Autodesk Fusion 360 part; units mm, degrees
(part 3 of 3)
sketch "DownZoneCables" plane through (0, 0, -18) normal (0, 0, -1) x (1, 0, 0)
  circle A0 centre (-23.3525, 0) radius 1.55
  circle A1 centre (23.3525, 0) radius 1.55
  arc A2 (-84.3286, -41.8567) -> (-84.3286, -41.2595) centre (-82.8076, -41.5581) ccw
  arc A3 (-84.3286, -41.2595) -> (-84.3286, -41.8567) centre (-84.3576, -41.5581) ccw
  arc A4 (87.6714, -41.8567) -> (87.6714, -41.2595) centre (89.1924, -41.5581) ccw
  arc A5 (87.6714, -41.2595) -> (87.6714, -41.8567) centre (87.6424, -41.5581) ccw
  arc A6 (-84.3286, 52.7522) -> (-84.3286, 53.3494) centre (-82.8076, 53.0508) ccw
  arc A7 (-84.3286, 53.3494) -> (-84.3286, 52.7522) centre (-84.3576, 53.0508) ccw
  arc A8 (87.6714, 52.7522) -> (87.6714, 53.3494) centre (89.1924, 53.0508) ccw
  arc A9 (87.6714, 53.3494) -> (87.6714, 52.7522) centre (87.6424, 53.0508) ccw
  arc A10 (84.2133, 53.3494) -> (84.2133, 52.7522) centre (82.6924, 53.0508) ccw
  arc A11 (84.2133, 52.7522) -> (84.2133, 53.3494) centre (84.2424, 53.0508) ccw
  arc A12 (1.4807, 16.7953) -> (1.9547, 17.1586) centre (2.6428, 15.7697) ccw
  arc A13 (1.9547, 17.1586) -> (1.4807, 16.7953) centre (1.7, 17) ccw
  arc A14 (-87.7867, -41.2595) -> (-87.7867, -41.8567) centre (-89.3076, -41.5581) ccw
  arc A15 (-87.7867, -41.8567) -> (-87.7867, -41.2595) centre (-87.7576, -41.5581) ccw
  arc A16 (-1.9531, 17.1611) -> (-1.4827, 16.7932) centre (-2.655, 15.7792) ccw
  arc A17 (-1.4827, 16.7932) -> (-1.9531, 17.1611) centre (-1.7, 17) ccw
  arc A18 (-87.7753, 53.3502) -> (-87.798, 52.7535) centre (-89.3065, 53.1098) ccw
  arc A19 (-87.798, 52.7535) -> (-87.7753, 53.3502) centre (-87.7576, 53.0508) ccw
  arc A20 (84.2133, -41.2595) -> (84.2133, -41.8567) centre (82.6924, -41.5581) ccw
  arc A21 (84.2133, -41.8567) -> (84.2133, -41.2595) centre (84.2424, -41.5581) ccw
  circle A22 centre (-107.5383, -7.4166) radius 1.55
  circle A23 centre (13.049, 34.0489) radius 1.55
  circle A24 centre (13.049, -34.7379) radius 1.55
  circle A25 centre (107.424, -7.4117) radius 1.55
  circle A26 centre (-13.049, 34.0489) radius 1.55
  circle A27 centre (-13.1642, -34.387) radius 1.55
  circle A28 centre (0, 0) radius 1.55
  line L0 (139, -65) -> (139, 64.9863)
  arc A29 (139, 64.9863) -> (130.116, 73.9855) centre (130, 64.9863) ccw
  spline S0 degree 3 poles (74.4883, 73.7463) (76.9901, 72.5973) (79.4645, 71.676) (81.9056, 70.9678) (87.9623, 69.2105) (93.8091, 68.7788) (99.3307, 68.9719) (104.8445, 69.1648) (110.025, 69.9298) (114.8797, 70.7875) (120.3191, 71.7486) (125.372, 72.8483) (130.116, 73.9855) knots -1 -1 -1 -1 -0.885821 -0.885821 -0.885821 -0.602514 -0.602514 -0.602514 -0.319613 -0.319613 -0.319613 -0.002638 -0.002638 -0.002638 -0.002638
  line L1 (74.4883, 73.7463) -> (74.1645, 73.895)
  arc A30 (74.1645, 73.895) -> (73.7471, 73.9863) centre (73.7471, 72.9863) ccw
  line L2 (73.7471, 73.9863) -> (-73.8561, 73.9863)
  arc A31 (-73.8561, 73.9863) -> (-74.2689, 73.8971) centre (-73.8561, 72.9863) ccw
  line L3 (-74.2689, 73.8971) -> (-74.6062, 73.7442)
  spline S1 degree 3 poles (-130.1182, 73.9855) (-125.3557, 72.8228) (-120.2812, 71.71) (-114.815, 70.7515) (-109.9113, 69.8915) (-104.6739, 69.1384) (-99.0955, 68.9821) (-93.5592, 68.8269) (-87.6968, 69.3115) (-81.6191, 71.1146) (-79.3104, 71.7996) (-76.9712, 72.6723) (-74.6062, 73.7442) knots 0.00269 0.00269 0.00269 0.00269 0.321768 0.321768 0.321768 0.608009 0.608009 0.608009 0.892088 0.892088 0.892088 1 1 1 1
  arc A32 (-130.1182, 73.9855) -> (-139, 64.9863) centre (-130, 64.9863) ccw
  line L4 (-139, 64.9863) -> (-139, -65)
  arc A33 (-139, -65) -> (-130, -74) centre (-130, -65) ccw
  line L5 (-130, -74) -> (130, -74)
  arc A34 (130, -74) -> (139, -65) centre (130, -65) ccw
  line L6 (-0.0576, -64.1328) -> (-85.2001, -64.455) construction
  line L7 (-120.0387, -64.455) -> (-85.2001, -64.455) construction
  line L8 (-120.0387, 64.6535) -> (-120.0387, -64.455) construction
  line L9 (107.424, 64.6535) -> (-120.0387, 64.6535) construction
  line L10 (107.424, -7.4117) -> (107.424, 64.6535) construction
  line L11 (-107.5383, -58.2757) -> (-77.6055, -58.2757) construction
  line L12 (-107.5383, -54.8501) -> (-107.5383, -58.2757) construction
  line L13 (-107.5383, -7.4166) -> (-107.5383, -54.8501) construction
  line L14 (-0.0576, -58.2757) -> (-77.6055, -58.2757) construction
  line L15 (-70.0576, 34.0489) -> (-70.0576, -52.4185) construction
  line L16 (-33.1654, 34.0489) -> (-70.0576, 34.0489) construction
  line L17 (-13.049, 34.0489) -> (-33.1654, 34.0489) construction
  line L18 (-0.0576, -52.4185) -> (-70.0576, -52.4185) construction
  line L19 (-64.1025, 27.0489) -> (-64.1025, -46.5614) construction
  line L20 (-33.1654, 27.0489) -> (-64.1025, 27.0489) construction
  line L21 (13.049, 27.0489) -> (-33.1654, 27.0489) construction
  line L22 (13.049, 34.0489) -> (13.049, 27.0489) construction
  line L23 (-0.0576, -46.5614) -> (-64.1025, -46.5614) construction
  line L24 (-58.5721, 14.3434) -> (-58.5721, -40.7043) construction
  line L25 (-33.329, 14.3434) -> (-58.5721, 14.3434) construction
  line L26 (0, 0) -> (-33.329, 14.3434) construction
  line L27 (-0.0576, -40.7043) -> (-58.5721, -40.7043) construction
  line L28 (-89.3076, -41.5581) -> (-89.3076, -48.5863) construction
  line L29 (-89.3076, -48.5863) -> (-76.4539, -48.5863) construction
  line L30 (-76.4539, 39.6391) -> (31.271, 39.6391) construction
  line L31 (31.271, 39.6391) -> (31.271, 21.1451) construction
  line L32 (31.271, 21.1451) -> (-2.7267, 21.1451) construction
  line L33 (-2.7267, 21.1451) -> (-2.655, 15.7792) construction
  line L34 (-76.4539, -48.5863) -> (-76.4539, 39.6391) construction
  line L35 (59.1924, -69) -> (59.1924, 46.7769) construction
  line L36 (59.1924, 46.7769) -> (-82.8076, 46.7769) construction
  line L37 (-82.8076, 46.7769) -> (-82.8076, -41.5581) construction
  line L38 (-89.3065, 53.1098) -> (-89.3075, 59.048) construction
  line L39 (-89.3075, 59.048) -> (89.1924, 59.0769) construction
  line L40 (89.1924, 59.0769) -> (89.1924, 53.0508) construction
  line L41 (89.1924, 53.0508) -> (89.1924, -41.5581) construction
  line L42 (-89.3076, -41.5581) -> (-89.3065, 53.1098) construction
  line L43 (66.6924, 53.0508) -> (66.6924, -69) construction
  line L44 (-82.8076, 53.0508) -> (66.6924, 53.0508) construction
  line L45 (74.1924, 52.9097) -> (81.6845, 52.9097) construction
  line L46 (74.1924, -69) -> (74.1924, 52.9097) construction
  line L47 (51.6924, 15.7697) -> (2.6428, 15.7697) construction
  line L48 (51.6924, -69) -> (51.6924, 15.7697) construction
  line L49 (81.6924, -69) -> (81.6924, -41.5581) construction
  line L50 (89.1924, -41.5581) -> (89.1924, -69) construction
  line L51 (35.9424, -69.99) -> (35.9424, -39.7739) construction
  line L52 (35.9424, -39.7739) -> (13.0118, -39.7739) construction
  line L53 (13.0118, -39.7739) -> (-0.0576, -34.8471) construction
  line L54 (-0.0576, -40.7043) -> (11.9424, -44.0082) construction
  line L55 (29.9424, -69.99) -> (29.9424, -44.8099) construction
  line L56 (11.9424, -44.0082) -> (29.9424, -44.8099) construction
  line L57 (23.9424, -69.99) -> (23.9424, -49.8459) construction
  line L58 (-0.0576, -46.5614) -> (23.9424, -49.8459) construction
  line L59 (17.9424, -69.99) -> (17.9424, -54.8819) construction
  line L60 (-0.0576, -52.4185) -> (17.9424, -54.8819) construction
  line L61 (11.9424, -69.99) -> (11.9424, -59.9179) construction
  line L62 (-0.0576, -58.2757) -> (11.9424, -59.9179) construction
  line L63 (5.9424, -69.99) -> (5.9424, -64.954) construction
  line L64 (-0.0576, -64.1328) -> (5.9424, -64.954) construction
  line L65 (53.2424, -69) -> (53.2424, 17.3197)
  line L66 (53.2424, 17.3197) -> (2.6428, 17.3197)
  line L67 (50.1424, -69) -> (50.1424, 14.2197)
  line L68 (50.1424, 14.2197) -> (2.6428, 14.2197)
  line L69 (60.7424, -69) -> (60.7424, 48.3269)
  line L70 (60.7424, 48.3269) -> (-84.3576, 48.3269)
  line L71 (-84.3576, 48.3269) -> (-84.3576, -41.5581)
  line L72 (-82.8076, 51.5008) -> (65.1424, 51.5008)
  line L73 (65.1424, 51.5008) -> (65.1424, -69)
  line L74 (75.7424, -69) -> (75.7424, 51.3597)
  line L75 (75.7424, 51.3597) -> (81.6845, 51.3597)
  line L76 (90.7424, -41.5581) -> (90.7424, -69)
  line L77 (90.7424, 53.0508) -> (90.7424, -41.5581)
  line L78 (90.7424, 60.6272) -> (90.7424, 53.0508)
  line L79 (-90.8577, 60.5977) -> (90.7424, 60.6272)
  line L80 (-90.8565, 53.1097) -> (-90.8577, 60.5977)
  line L81 (-90.8576, -41.5581) -> (-90.8565, 53.1097)
  line L82 (-90.8576, -41.5581) -> (-90.8576, -50.1363)
  line L83 (-90.8576, -50.1363) -> (-74.9039, -50.1363)
  line L84 (-74.9039, -50.1363) -> (-74.9039, 38.0891)
  line L85 (-74.9039, 38.0891) -> (29.721, 38.0891)
  line L86 (29.721, 38.0891) -> (29.721, 22.6951)
  line L87 (29.721, 22.6951) -> (-4.2976, 22.6951)
  line L88 (-4.2976, 22.6951) -> (-4.2049, 15.7584)
  line L89 (-1.1559, 19.5951) -> (-1.1051, 15.7999)
  line L90 (32.821, 19.5951) -> (-1.1559, 19.5951)
  line L91 (32.821, 41.1891) -> (32.821, 19.5951)
  line L92 (-78.0039, 41.1891) -> (32.821, 41.1891)
  line L93 (-78.0039, -47.0363) -> (-78.0039, 41.1891)
  line L94 (-87.7576, -47.0363) -> (-78.0039, -47.0363)
  line L95 (-87.7576, -41.5581) -> (-87.7576, -47.0363)
  line L96 (-87.7576, -41.5581) -> (-87.7565, 53.1099)
  line L97 (-87.7565, 53.1099) -> (-87.7572, 57.4982)
  line L98 (-87.7572, 57.4982) -> (87.6424, 57.5267)
  line L99 (87.6424, 57.5267) -> (87.6424, 53.0508)
  line L100 (87.6424, 53.0508) -> (87.6424, -41.5581)
  line L101 (87.6424, -41.5581) -> (87.6424, -69)
  line L102 (80.1424, -69) -> (80.1424, -41.5581)
  line L103 (72.6424, -69) -> (72.6424, 54.4597)
  line L104 (72.6424, 54.4597) -> (81.6845, 54.4597)
  line L105 (108.974, -7.4117) -> (108.974, 66.2035)
  line L106 (108.974, 66.2035) -> (-121.5887, 66.2035)
  line L107 (-121.5887, 66.2035) -> (-121.5887, -66.005)
  line L108 (-121.5887, -66.005) -> (-85.1972, -66.005)
  line L109 (-0.2303, -65.6835) -> (-85.1972, -66.005)
  line L110 (-0.0576, -56.7257) -> (-77.6055, -56.7257)
  line L111 (-105.9883, -56.7257) -> (-77.6055, -56.7257)
  line L112 (-105.9883, -54.8501) -> (-105.9883, -56.7257)
  line L113 (-105.9883, -7.4166) -> (-105.9883, -54.8501)
  line L114 (-0.0576, -50.8685) -> (-68.5076, -50.8685)
  line L115 (-68.5076, 32.4989) -> (-68.5076, -50.8685)
  line L116 (-33.1654, 32.4989) -> (-68.5076, 32.4989)
  line L117 (-13.049, 32.4989) -> (-33.1654, 32.4989)
  line L118 (-0.0576, -39.1543) -> (-57.0221, -39.1543)
  line L119 (-57.0221, 12.7934) -> (-57.0221, -39.1543)
  line L120 (-33.6484, 12.7934) -> (-57.0221, 12.7934)
  line L121 (-0.6127, -1.4238) -> (-33.6484, 12.7934)
  line L122 (0.1238, -42.3619) -> (11.6991, -45.5489)
  line L123 (11.6991, -45.5489) -> (28.3924, -46.2924)
  line L124 (28.3924, -69.99) -> (28.3924, -46.2924)
  line L125 (0.1067, -54.0055) -> (16.3924, -56.2343)
  line L126 (16.3924, -69.99) -> (16.3924, -56.2343)
  line L127 (0.0055, -59.8488) -> (10.3924, -61.2703)
  line L128 (10.3924, -69.99) -> (10.3924, -61.2703)
  line L129 (-0.0909, -65.6927) -> (4.3924, -66.3063)
  line L130 (4.3924, -69.99) -> (4.3924, -66.3063)
  line L131 (35.9424, -69.99) -> (35.9424, -39.7739) construction
  line L132 (35.9424, -39.7739) -> (13.0118, -39.7739) construction
  line L133 (13.0118, -39.7739) -> (-0.0576, -34.8471) construction
  line L134 (-0.0576, -40.7043) -> (11.9424, -44.0082) construction
  line L135 (29.9424, -69.99) -> (29.9424, -44.8099) construction
  line L136 (11.9424, -44.0082) -> (29.9424, -44.8099) construction
  line L137 (23.9424, -69.99) -> (23.9424, -49.8459) construction
  line L138 (-0.0576, -46.5614) -> (23.9424, -49.8459) construction
  line L139 (17.9424, -69.99) -> (17.9424, -54.8819) construction
  line L140 (-0.0576, -52.4185) -> (17.9424, -54.8819) construction
  line L141 (11.9424, -69.99) -> (11.9424, -59.9179) construction
  line L142 (-0.0576, -58.2757) -> (11.9424, -59.9179) construction
  line L143 (5.9424, -69.99) -> (5.9424, -64.954) construction
  line L144 (-0.0576, -64.1328) -> (5.9424, -64.954) construction
  line L145 (57.6424, -69) -> (57.6424, 45.2269)
  line L146 (57.6424, 45.2269) -> (-81.2576, 45.2269)
  line L147 (-81.2576, 45.2269) -> (-81.2576, -41.5581)
  line L148 (-82.8076, 54.6008) -> (68.2424, 54.6008)
  line L149 (68.2424, 54.6008) -> (68.2424, -69)
  line L150 (105.874, -7.4117) -> (105.874, 63.1035)
  line L151 (105.874, 63.1035) -> (-118.4887, 63.1035)
  line L152 (-118.4887, 63.1035) -> (-118.4887, -62.905)
  line L153 (-118.4887, -62.905) -> (-85.203, -62.905)
  line L154 (-0.0635, -62.5828) -> (-85.203, -62.905)
  line L155 (-109.0883, -7.4166) -> (-109.0883, -54.8501)
  line L156 (-109.0883, -54.8501) -> (-109.0883, -59.8257)
  line L157 (-109.0883, -59.8257) -> (-77.6055, -59.8257)
  line L158 (-0.3335, -59.8257) -> (-77.6055, -59.8257)
  line L159 (-0.4356, -53.9685) -> (-71.6076, -53.9685)
  line L160 (-71.6076, 35.5989) -> (-71.6076, -53.9685)
  line L161 (-33.1654, 35.5989) -> (-71.6076, 35.5989)
  line L162 (-13.049, 35.5989) -> (-33.1654, 35.5989)
  line L163 (0.6127, 1.4238) -> (-33.0097, 15.8934)
  line L164 (-33.0097, 15.8934) -> (-60.1221, 15.8934)
  line L165 (-60.1221, 15.8934) -> (-60.1221, -42.2543)
  line L166 (-0.6726, -42.2543) -> (-60.1221, -42.2543)
  line L167 (0.1525, -62.5971) -> (7.4924, -63.6016)
  line L168 (7.4924, -69.99) -> (7.4924, -63.6016)
  line L169 (0.1525, -56.74) -> (13.4924, -58.5656)
  line L170 (13.4924, -69.99) -> (13.4924, -58.5656)
  line L171 (0.1525, -50.8829) -> (19.4924, -53.5296)
  line L172 (19.4924, -69.99) -> (19.4924, -53.5296)
  line L173 (0.3538, -39.2099) -> (12.1856, -42.4675)
  line L174 (12.1856, -42.4675) -> (31.4924, -43.3274)
  line L175 (31.4924, -69.99) -> (31.4924, -43.3274)
  line L176 (0.3538, -39.2099) -> (-0.0576, -39.1543)
  line L177 (4.3924, -69.99) -> (7.4924, -69.99)
  line L178 (10.3924, -69.99) -> (13.4924, -69.99)
  line L179 (16.3924, -69.99) -> (19.4924, -69.99)
  line L180 (28.3924, -69.99) -> (31.4924, -69.99)
  line L181 (34.3924, -69.99) -> (37.4924, -69.99)
  line L182 (50.1424, -69) -> (53.2424, -69)
  line L183 (57.6424, -69) -> (60.7424, -69)
  line L184 (65.1424, -69) -> (68.2424, -69)
  line L185 (72.6424, -69) -> (75.7424, -69)
  line L186 (80.1424, -69) -> (83.2424, -69)
  line L187 (87.6424, -69) -> (90.7424, -69)
  line L188 (105.874, -7.4117) -> (108.974, -7.4117)
  line L189 (81.6845, 54.4597) -> (81.6845, 51.3597)
  line L190 (-0.6127, -1.4238) -> (0.6127, 1.4238)
  line L191 (2.6428, 14.2197) -> (2.6428, 17.3197)
  line L192 (-1.1051, 15.7999) -> (-4.2049, 15.7584)
  line L193 (-13.049, 32.4989) -> (-13.049, 35.5989)
  line L194 (-81.2576, -41.5581) -> (-84.3576, -41.5581)
  line L195 (-82.8076, 51.5008) -> (-82.8076, 54.6008)
  line L196 (-105.9883, -7.4166) -> (-109.0883, -7.4166)
  line L197 (-0.6044, -36.2975) -> (0.4891, -33.3967)
  line L198 (-0.0576, -50.8685) -> (0.1525, -50.8829)
  line L199 (-0.0576, -56.7257) -> (0.1525, -56.74)
  line L200 (-0.0635, -62.5828) -> (0.1525, -62.5971)
  arc A35 (-0.0909, -65.6927) -> (-0.2303, -65.6835) centre (-0.2265, -66.6835) ccw
  arc A36 (0.0055, -59.8488) -> (-0.3335, -59.8257) centre (-0.3335, -62.3257) ccw
  arc A37 (0.1067, -54.0055) -> (-0.4356, -53.9685) centre (-0.4356, -57.9685) ccw
  arc A38 (0.1238, -42.3619) -> (-0.6726, -42.2543) centre (-0.6726, -45.2543) ccw
  line L201 (-0.0576, -45.0114) -> (-62.5525, -45.0114)
  line L202 (-62.5525, 25.4989) -> (-62.5525, -45.0114)
  line L203 (-33.1654, 25.4989) -> (-62.5525, 25.4989)
  line L204 (14.599, 25.4989) -> (-33.1654, 25.4989)
  line L205 (14.599, 34.0489) -> (14.599, 25.4989)
  line L206 (-0.0576, -48.1114) -> (-65.6525, -48.1114)
  line L207 (-65.6525, 28.5989) -> (-65.6525, -48.1114)
  line L208 (-33.1654, 28.5989) -> (-65.6525, 28.5989)
  line L209 (11.499, 28.5989) -> (-33.1654, 28.5989)
  line L210 (11.499, 34.0489) -> (11.499, 28.5989)
  line L211 (11.499, 34.0489) -> (14.599, 34.0489)
  line L212 (0.1525, -45.0257) -> (25.4924, -48.4936)
  line L213 (25.4924, -69.99) -> (25.4924, -48.4936)
  line L214 (-0.2678, -48.0971) -> (22.3924, -51.1982)
  line L215 (22.3924, -69.99) -> (22.3924, -51.1982)
  line L216 (-0.0576, -45.0114) -> (0.1525, -45.0257)
  line L217 (22.3924, -69.99) -> (25.4924, -69.99)
  line L218 (-0.0576, -28.99) -> (13.049, -28.99) construction
  line L219 (13.049, -28.99) -> (13.049, -34.7379) construction
  line L220 (41.9424, -34.7379) -> (13.049, -34.7379) construction
  line L221 (41.9424, -69.99) -> (41.9424, -34.7379) construction
  line L222 (-0.0576, -30.54) -> (11.499, -30.54)
  line L223 (11.499, -30.54) -> (11.499, -36.2879)
  line L224 (40.3924, -36.2879) -> (11.499, -36.2879)
  line L225 (40.3924, -69.99) -> (40.3924, -36.2879)
  line L226 (43.4924, -69.99) -> (43.4924, -33.1879)
  line L227 (43.4924, -33.1879) -> (14.599, -33.1879)
  line L228 (14.599, -27.44) -> (14.599, -33.1879)
  line L229 (-0.0576, -27.44) -> (14.599, -27.44)
  line L230 (40.3924, -69.99) -> (43.4924, -69.99)
  line L231 (-0.0576, -30.54) -> (-0.0576, -27.44)
  line L232 (-0.0576, -34.8471) -> (-13.1642, -34.387) construction
  line L233 (37.4924, -69.99) -> (37.4924, -38.2239)
  line L234 (37.4924, -38.2239) -> (13.2942, -38.2239)
  line L235 (13.2942, -38.2239) -> (0.251, -33.307)
  line L236 (0.251, -33.307) -> (-13.1098, -32.8379)
  line L237 (34.3924, -69.99) -> (34.3924, -41.3239)
  line L238 (34.3924, -41.3239) -> (12.7293, -41.3239)
  line L239 (12.7293, -41.3239) -> (-0.3663, -36.3872)
  line L240 (-0.3663, -36.3872) -> (-13.2186, -35.936)
  line L241 (-13.1098, -32.8379) -> (-13.2186, -35.936)
  line L242 (84.0907, -42.2268) -> (83.2424, -45.6976)
  line L243 (81.7844, -40.1809) -> (80.1424, -41.5581)
  line L244 (81.7844, -40.1809) -> (84.0907, -42.2268)
  line L245 (83.2424, -69) -> (83.2424, -45.6976)
  dimension "d158" = 1.55
  dimension "d160" = 1.55
  dimension "d161" = 1.55
  dimension "d162" = 1.55
  dimension "d164" = 1.55
  dimension "d165" = 1.55
  dimension "d169" = 1.55
  dimension "d170" = 1.55
  dimension "d172" = 1.55
  dimension "d173" = 1.55
  dimension "d186" = 1.55
  dimension "d192" = 1
  dimension "d193" = 2.5
  dimension "d194" = 4
  dimension "d197" = 3
  constraint vertical L22
  constraint perpendicular L21 L22
  constraint parallel L17 L21
  constraint vertical L10
  constraint perpendicular L9 L10
  constraint perpendicular L8 L9
  constraint perpendicular L7 L8
  constraint vertical L13
  constraint perpendicular L28 L29
  constraint perpendicular L29 L34
  constraint perpendicular L28 L30
  constraint perpendicular L29 L31
  constraint perpendicular L31 L32
  constraint perpendicular L15 L16
  constraint parallel L20 L21
  constraint perpendicular L19 L21
  constraint horizontal L25
  constraint perpendicular L24 L25
  constraint perpendicular L24 L27
  constraint perpendicular L19 L23
  constraint perpendicular L15 L18
  constraint perpendicular L12 L14
  constraint perpendicular L11 L12
  constraint vertical L49
  constraint perpendicular L45 L46
  constraint perpendicular L44 L46
  constraint perpendicular L43 L44
  constraint perpendicular L30 L35
  constraint perpendicular L36 L37
  constraint perpendicular L47 L48
  constraint perpendicular L38 L39
  constraint vertical L40
  constraint vertical L63
  constraint parallel L61 L63
  constraint parallel L59 L61
  constraint parallel L57 L59
  constraint parallel L55 L57
  constraint perpendicular L51 L52
  constraint vertical L143
  constraint parallel L141 L143
  constraint parallel L139 L141
  constraint parallel L137 L139
  constraint parallel L135 L137
  constraint perpendicular L131 L132
  constraint perpendicular L130 L177
  constraint perpendicular L130 L178
  constraint perpendicular L172 L179
  constraint perpendicular L175 L180
  constraint perpendicular L51 L181
  constraint perpendicular L65 L182
  constraint perpendicular L35 L183
  constraint perpendicular L149 L184
  constraint perpendicular L74 L185
  constraint perpendicular L186 L245
  constraint perpendicular L76 L187
  constraint perpendicular L105 L188
  constraint perpendicular L75 L189
  constraint perpendicular L163 L190
  constraint perpendicular L66 L191
  constraint perpendicular L88 L192
  constraint perpendicular L17 L193
  constraint coincident A3.centre L71.end
  constraint perpendicular L71 L194
  constraint perpendicular L148 L195
  constraint perpendicular L155 L196
  constraint perpendicular L197 L235
  constraint parallel L10 L105
  constraint parallel L9 L106
  constraint parallel L8 L107
  constraint parallel L7 L108
  constraint parallel L6 L109
  constraint parallel L64 L129
  constraint parallel L63 L130
  constraint tangent L109 A35
  constraint tangent L129 A35
  constraint parallel L62 L127
  constraint parallel L61 L128
  constraint parallel L13 L155
  constraint parallel L12 L156
  constraint parallel L11 L157
  constraint parallel L14 L158
  constraint tangent L127 A36
  constraint tangent L158 A36
  constraint parallel L60 L125
  constraint parallel L59 L126
  constraint parallel L18 L159
  constraint parallel L15 L160
  constraint parallel L16 L161
  constraint parallel L17 L162
  constraint tangent L125 A37
  constraint tangent L159 A37
  constraint parallel L54 L122
  constraint parallel L56 L123
  constraint parallel L55 L124
  constraint parallel L26 L163
  constraint parallel L25 L164
  constraint parallel L24 L165
  constraint parallel L27 L166
  constraint tangent L122 A38
  constraint tangent L166 A38
  constraint perpendicular L205 L211
  constraint perpendicular L213 L217
  constraint perpendicular L218 L219
  constraint parallel L219 L221
  constraint perpendicular L219 L220
  constraint perpendicular L221 L230
  constraint perpendicular L218 L231
  constraint coincident A27.centre L232.end
  constraint perpendicular L236 L241
  constraint coincident A20 L242.start
  constraint parallel L49 L245
  measures "d192" radius of A35
  measures "d193" radius of A36
  measures "d194" radius of A37
  measures "d197" radius of A38
extrude "Extrude13" cut sketch "DownZoneCables" against normal blind 3 contours A2 A3 L69 L70 L71 L145 L146 L147 L183 | A4 A5 L76 L101 L187 | A4 A5 A8 A9 L77 L100 | A8 A9 A18 A19 L78 L79 L80 L97 L98 L99 | A14 A15 A18 A19 L81 L96 | A14 A15 A16 A17 L82 L83 L84 L85 L86 L87 L88 L89 L90 L91 L92 L93 L94 L95 | A6 L72 L73 L148 L149 L184 | A10 L74 L75 L103 L104 L185 L189 | A12 L65 L66 L67 L68 L182 | A20 L102 L186 L242 L243 L244 L245 | A22 L110 L111 L112 L113 L127 L128 L155 L156 L157 L158 L169 L170 L178 L199 A36 | A23 L201 L202 L203 L204 L205 L206 L207 L208 L209 L210 L212 L213 L214 L215 L216 L217 | A24 L222 L223 L224 L225 L226 L227 L228 L229 L230 L231 | A25 L105 L106 L107 L108 L109 L129 L130 L150 L151 L152 L153 L154 L167 L168 L177 L200 A35 | A26 L114 L115 L116 L117 L125 L126 L159 L160 L161 L162 L171 L172 L179 L198 A37 | A27 L241 | A27 L181 L233 L234 L235 L236 L237 L238 L239 L240 | A28 L118 L119 L120 L121 L122 L123 L124 L163 L164 L165 L166 L173 L174 L175 L176 L180 A38 picked at (-12.6694, -34.5357) bodies 2
extrude "Extrude14" cut sketch "Cable Management" against normal blind 4 contours L21 A6 A14 L40 L44 | L21 A19 | L21 A6 A14 L40 L43 | A6 A14 A18 | L41 A16 L42 A17 | A20 L46 L47 A21 | A22 L48 L49 A23 | A24 L50 L51 A25 | A26 L52 L53 A27 | A28 L54 L55 A29 | A30 L56 L57 A31 | A32 L58 L59 A33 | A34 L60 A35 L61 | A36 L62 A37 L63 | A38 L64 A39 L65 | A40 L66 A41 L67 | A42 L71 A43 L72 bodies 2
extrude "Extrude15" add sketch "Cable Management" along normal blind 5 separate body contours A6 A7 L36 L37 A18 | A6 A14 A18 | A7 A8 L36 L37 | A7 | A8 A9 L36 L37 | A8 | A9 A10 L36 L37 | A9 | A10 A11 L36 L37 | A10 | A11 A12 L36 L37 | A11 | A12 A13 L36 L37 | A12 | A13 A15 makes body 10
move_body "Move11" bodies 10 to x (1, 0, 0) y (0, 1, 0) z (0, 0, 1) at (0, 0, 18)
combine "Combine3" operation cut target body 2 tool bodies 10
extrude "Extrude16" cut sketch "Cable Management" against normal blind 18 contours A6 A14 A18 | A7 | A8 | A9 | A10 | A11 | A12 | A13 A15 bodies 2
copy_body "CopyPasteBodies6" bodies 2 makes body 11
move_body "Move7" bodies 11 to x (-1, 0, 0) y (0, 1, 0) z (0, 0, -1) at (278, 0, -2)
move_body "Move8" bodies 11 to x (1, 0, 0) y (0, 1, 0) z (0, 0, 1) at (0, 0, -17)
move_body "Move9" bodies 11 to x (1, 0, 0) y (0, 1, 0) z (0, 0, 1) at (20, 0, 0)
extrude "Extrude17" add sketch "CutAround" against normal blind 18 separate body contours L10 A6 L11 A7 L12 S2 A8 L13 A9 L14 A10 L15 A11 S3 makes body 12
extrude "Extrude18" cut sketch "RefPoints" against normal blind 18 contours A11 | A12 bodies 12
move_body "Move12" bodies 12 to x (1, 0, 0) y (0, 1, 0) z (0, 0, 1) at (-298, 0, 1)
equation "BitSize = 3 mm"
equation "BitSizeWithMarge = 3.1 mm"
equation "SolderingPit = 8 mm"
equation "WoodHeight = 18 mm"
equation "d68 = -WoodHeight"
equation "d75 = BitSizeWithMarge"
equation "d76 = BitSizeWithMarge"
equation "d77 = BitSizeWithMarge"
equation "d78 = BitSizeWithMarge"
equation "d79 = BitSizeWithMarge"
equation "d80 = BitSizeWithMarge"
equation "d81 = BitSizeWithMarge"
equation "d82 = BitSizeWithMarge"
equation "d83 = BitSizeWithMarge"
equation "d84 = BitSizeWithMarge"
equation "d85 = -WoodHeight"
equation "d91 = -WoodHeight"
equation "d109 = BitSizeWithMarge"
equation "d110 = BitSizeWithMarge"
equation "d120 = -WoodHeight"
equation "d130 = -WoodHeight"
equation "d139 = BitSizeWithMarge"
equation "d144 = BitSizeWithMarge"
equation "d146 = BitSizeWithMarge"
equation "d147 = BitSizeWithMarge"
equation "TunnelHalfSize = BitSizeWithMarge / 2"
equation "d158 = TunnelHalfSize"
equation "d159 = -TunnelHalfSize"
equation "d160 = TunnelHalfSize"
equation "d161 = TunnelHalfSize"
equation "d162 = TunnelHalfSize"
equation "d164 = TunnelHalfSize"
equation "d165 = TunnelHalfSize"
equation "d166 = -TunnelHalfSize"
equation "d167 = -TunnelHalfSize"
equation "d169 = TunnelHalfSize"
equation "d170 = TunnelHalfSize"
equation "d172 = TunnelHalfSize"
equation "d173 = TunnelHalfSize"
equation "d179 = -TunnelHalfSize"
equation "d180 = -TunnelHalfSize"
equation "d181 = -TunnelHalfSize"
equation "d186 = TunnelHalfSize"
equation "d187 = -TunnelHalfSize"
equation "d188 = -TunnelHalfSize"
equation "d190 = -TunnelHalfSize"
equation "d191 = -TunnelHalfSize"
equation "d198 = -TunnelHalfSize"
equation "d199 = -TunnelHalfSize"
equation "d200 = -TunnelHalfSize"
equation "d201 = --TunnelHalfSize"
equation "d203 = -TunnelHalfSize"
equation "d204 = -TunnelHalfSize"
equation "d213 = WoodHeight"
equation "d214 = WoodHeight * -1"
equation "d216 = WoodHeight * -1"
equation "d218 = -WoodHeight"
named bodies: "LightResistor", "woodboard", "LightResistor (1)", "LightResistor (2)", "LightResistor (3)", "LightResistor (4)", "woodboard (1)", "WoodboardCutAround"
